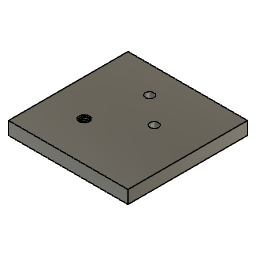
GVS011 mounting plate (Autodesk Fusion 360 design; units mm, degrees)
Autodesk Fusion 360 part; units mm, degrees
box "BoxPrimitive1" add length 46.228 width 46.228 height 5.0038 placed x (0, 1, 0) y (-1, 0, 0) z (0, 0, 1) at (46.228, 0, 0) makes body 1
cylinder "CylinderPrimitive2" add diameter 4.572 height 5.0038 placed x (1, 0, 0) y (0, 1, 0) z (0, 0, 1) at (0, 0, 0) separate body makes body 2
move_body "Move5" bodies 2 to x (1, 0, 0) y (0, 1, 0) z (0, 0, 1) at (14.224, 14.224, 0)
cylinder "CylinderPrimitive3" add diameter 3.302 height 5.0038 placed x (1, 0, 0) y (0, 1, 0) z (0, 0, 1) at (0, 0, 0) separate body makes body 3
move_body "Move6" bodies 3 to x (1, 0, 0) y (0, 1, 0) z (0, 0, 1) at (29.718, 26.67, 0)
cylinder "CylinderPrimitive4" add diameter 3.302 height 5.0038 placed x (1, 0, 0) y (0, 1, 0) z (0, 0, 1) at (0, 0, 0) separate body makes body 4
move_body "Move7" bodies 4 to x (1, 0, 0) y (0, 1, 0) z (0, 0, 1) at (18.796, 35.814, 0)
move_body "Move8" bodies 2 to x (1, 0, 0) y (0, 1, 0) z (0, 0, 1) at (0, 1.016, 0)
combine "Combine5" operation cut target body 1 tool bodies 2
combine "Combine6" operation cut target body 1 tool bodies 4
combine "Combine7" operation cut target body 1 tool bodies 3
thread "Thread5" "ANSI Unified Screw Threads 0.164(#8) 8-32 UNC 3B" major diameter 4.1656 minor diameter 3.4163 pitch 0.7937 angle 60 modelled right hand crest width 0.2414 on face at (16.4986, 15.0124, 3.3359) crest through (15.9322, 15.24, 0.1984) on bodies 1
